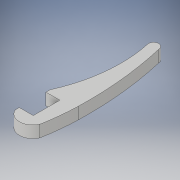
# Autodesk Inventor part: leg
Saved by Autodesk Inventor 2018 (Build 220112000, 112)
## iProperties
Created: 2017-12-28
Part Number: leg
Material: Generic
Document SubType Name: Modeling
Designer: BB-8
Density: 1 g/cm^3
Appearance: Default
Author: BB-8
Autodesk Inventor part; units mm, degrees
ref_plane "YZ Plane" through (0, 0, 0) normal (1, 0, 0) x (0, 1, 0)
ref_plane "XZ Plane" through (0, 0, 0) normal (0, 1, 0) x (-1, 0, 0)
ref_plane "XY Plane" through (0, 0, 0) normal (0, 0, 1) x (1, 0, 0)
sketch "Sketch2" plane through (0, 0, 0) normal (0, 1, 0) x (-1, 0, 0)
  line L0 (0, 0) -> (11.8, 0)
  line L1 (11.8, 16.9404) -> (11.8, 22.5)
  line L2 (11.8, 22.5) -> (0, 22.5)
  line L3 (0, 22.5) -> (0, 0)
  arc A0 (-9.1414, 25.9755) -> (-12.2, -3.5) centre (181.3562, -8.6883) ccw
  arc A1 (11.8, 26) -> (-9.1414, 25.9755) centre (1.3346, 21.4702) ccw
  arc A2 (-4.4957, -79) -> (3.7221, -77.2478) centre (-0.2, -79) ccw
  arc A3 (-12.2, -3.5) -> (-4.4957, -79) centre (283.8313, -11.4351) ccw
  arc A4 (11.8, -3.5) -> (4.0957, -79) centre (122.1776, -52.9064) ccw
  line L4 (11.8, -3.5) -> (11.8, 0)
  line L5 (11.8, 22.5) -> (11.8, 26)
  dimension "d2" = 11.8
  dimension "d3" = 22.5
  constraints: 13 point on circle, 12 end point, 5 centre point, 2 parallel, 1 horizontal, 1 perpendicular, 1 point on line, 1 tangent
  measures "d2" distance of L2.end L1.end
  measures "d3" distance of L1.end L0.end
extrude "Extrusion1" add sketch "Sketch2" along normal blind 10 contours L0 L4 A4 A2 A3 A0 A1 L5 L2 L3
body "Solid1"
